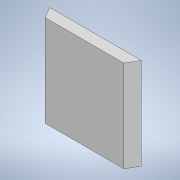
# Autodesk Inventor part: SatelliteSideWallFilled_v2
Saved by Autodesk Inventor 2020 (Build 240168000, 168)
## iProperties
Created: 2020-03-05
Part Number: SatelliteSideWallFilled_v2
Material: Generic
Document SubType Name: Modeling
Designer: WANG
Density: 1 g/cm^3
Appearance: Default
Author: WANG
Autodesk Inventor part; units mm, degrees
ref_plane "YZ Plane" through (0, 0, 0) normal (1, 0, 0) x (0, 1, 0)
ref_plane "XZ Plane" through (0, 0, 0) normal (0, 1, 0) x (-1, 0, 0)
ref_plane "XY Plane" through (0, 0, 0) normal (0, 0, 1) x (1, 0, 0)
sketch "Sketch1" plane through (0, 0, 0) normal (0, 1, 0) x (-1, 0, 0)
  line L0 (-107.95, -0.0035) -> (-53.978, 93.4857)
  line L1 (-53.978, 93.4857) -> (53.972, 93.4892)
  line L2 (53.972, 93.4892) -> (107.95, 0.0035)
  line L3 (107.95, 0.0035) -> (53.978, -93.4857)
  line L4 (53.978, -93.4857) -> (-53.972, -93.4892)
  line L5 (-53.972, -93.4892) -> (-107.95, -0.0035)
  line L6 (-92.964, 0.0336) -> (-46.4529, 80.526)
  line L7 (-46.4529, 80.526) -> (46.5111, 80.4924)
  line L8 (46.5111, 80.4924) -> (92.964, -0.0336)
  line L9 (92.964, -0.0336) -> (46.4529, -80.526)
  line L10 (46.4529, -80.526) -> (-46.5111, -80.4924)
  line L11 (-46.5111, -80.4924) -> (-92.964, 0.0336)
  line L12 (53.978, -93.4857) -> (46.4529, -80.526)
  line L13 (-53.972, -93.4892) -> (-46.5111, -80.4924)
  point P0 (0, 0)
  point P1 (0, 0)
  point P2 (0, 0)
  point P3 (0, 0)
  dimension "d0" = 215.9
  dimension "d1" = 14.986
  constraints: 28 end point, 2 coincident, 26 other
  measures "d0" distance of L0.start L2.end
  measures "d1" distance of L0.start L6.start
extrude "Extrusion1" add sketch "Sketch1" along normal blind 107.95 contours L13 L10 L12 L4
body "Solid1"
